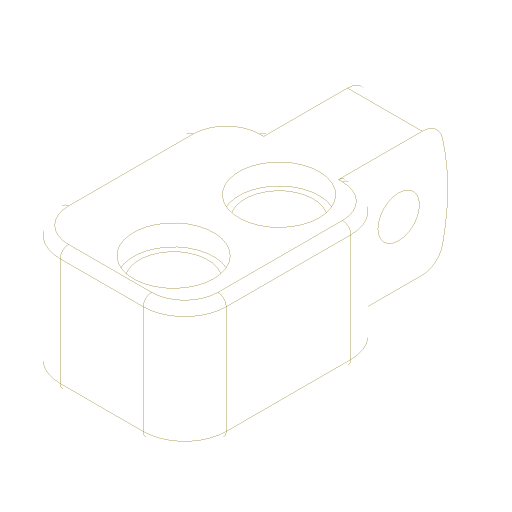
# Autodesk Inventor part: Camera_holder_PCB_1DOF
Saved by Autodesk Inventor 2023 (Build 270158000, 158)
## iProperties
Created: 2024-06-13
Part Number: Camera_holder_PCB_1DOF
Material: Generic
Document SubType Name: Modeling
Designer: ferrerx
Density: 1 g/cm^3
Appearance: Nylon 6
Author: ferrerx
Autodesk Inventor part; units mm, degrees
ref_plane "YZ Plane" through (0, 0, 0) normal (1, 0, 0) x (0, 1, 0)
ref_plane "XZ Plane" through (0, 0, 0) normal (0, 1, 0) x (-1, 0, 0)
ref_plane "XY Plane" through (0, 0, 0) normal (0, 0, 1) x (1, 0, 0)
sketch "Sketch1" plane through (0, 0, 0) normal (0, 1, 0) x (-1, 0, 0)
  line L0 (-2, 2.5) -> (2, 2.5)
  line L1 (2, 2.5) -> (2, -2.5)
  line L2 (2, -2.5) -> (-2, -2.5)
  line L3 (-2, -2.5) -> (-2, 2.5)
  line L4 (-2, 2.5) -> (2, -2.5) construction
  line L5 (2, 2.5) -> (-2, -2.5) construction
  line L6 (0, 0) -> (2, 0) construction
  circle A0 centre (-0.5, 1.27) radius 0.825
  line L7 (-0.5, 1.27) -> (-0.5, 0) construction
  circle A1 centre (-0.5, -1.27) radius 0.825
  line L8 (-0.5, -1.27) -> (-0.5, 0) construction
  dimension "d0" = 4
  dimension "d1" = 5
  dimension "d3" = 1.65
  dimension "d4" = 1.27
  dimension "d5" = 1.5
  constraints: 18 end point, 3 midpoint, 2 centre point, 2 parallel, 1 horizontal, 1 perpendicular, 1 symmetric about line, 1 vertical, 1 other
  measures "d0" distance of L1.end L2.end
  measures "d1" distance of L0.end L1.end
  measures "d3" diameter of A0
  measures "d4" distance from line of L6 L7.start
  measures "d5" distance between parallel lines of L3 L7
extrude "Extrusion1" add sketch "Sketch1" along normal blind 3
sketch "Sketch2" plane through (0, 3, 0) normal (0, 1, 0) x (1, 0, 0)
  circle A0 centre (0.5, -1.27) radius 0.825 projected
  circle A1 centre (0.5, -1.27) radius 0.965
  circle A2 centre (0.5, 1.27) radius 0.825 projected
  circle A3 centre (0.5, 1.27) radius 0.965
  point P0 (0, 0)
  dimension "d8" = 1.93
  dimension "d9" = 1.93
  constraints: 2 centre point, 2 coincident
  measures "d8" diameter of A1
  measures "d9" diameter of A3
extrude "Extrusion2" cut sketch "Sketch2" against normal blind 0.5
sketch "Sketch3" plane through (0, 3, 0) normal (0, 1, 0) x (1, 0, 0)
  line L0 (2, 2.5) -> (-2, 2.5) projected
  line L1 (-0.9, 2.5) -> (0.9, 2.5)
  line L2 (0.9, 2.5) -> (0.9, 5)
  line L3 (0.9, 5) -> (-0.9, 5)
  line L4 (-0.9, 5) -> (-0.9, 2.5)
  line L5 (-2, -2.5) -> (2, -2.5) projected
  line L6 (0, -2.5) -> (0, 2.5) construction
  point P0 (0, 0)
  dimension "d12" = 2.5
  dimension "d13" = 1.8
  constraints: 10 end point, 2 midpoint, 2 parallel, 1 horizontal, 1 perpendicular, 1 point on line, 1 vertical
  measures "d12" distance of L3.end L1.start
  measures "d13" distance between parallel lines of L2 L4
extrude "Extrusion3" add sketch "Sketch3" against normal up to surface (3 mm away)
sketch "Sketch4" plane through (0.9, 3, -2.5) normal (1, 0, 0) x (0, 0, -1)
  line L0 (2.2, 0) -> (2.2, -3) construction
  arc A0 (2.2, -3) -> (2.2, 0) centre (-2.5697, -1.5) ccw
  line L1 (2.5, 0) -> (2.5, -3) projected
  line L2 (2.2, 0) -> (2.5, 0)
  line L3 (2.5, 0) -> (2.5, -3)
  line L4 (2.5, -3) -> (2.2, -3)
  line L5 (2.5, -1.5) -> (1.25, -1.5) construction
  circle A1 centre (1.25, -1.5) radius 0.5
  point P0 (-2.5, -3)
  dimension "d16" = 5
  dimension "d17" = 0.3
  dimension "d18" = 1
  dimension "d19" = 1.25
  constraints: 10 end point, 2 centre point, 2 horizontal, 2 point on circle, 1 coincident, 1 collinear, 1 midpoint, 1 perpendicular, 1 vertical
  measures "d16" radius of A0
  measures "d17" distance between parallel lines of L0 L1
  measures "d18" diameter of A1
  measures "d19" distance of L5.start L5.end
extrude "Extrusion4" cut sketch "Sketch4" against normal blind 10
fillet "Fillet1" radius 0.5 2 edges at (0, 3, -4.7) (0, 0, -4.7)
fillet "Fillet2" radius 1 4 edges at (2, 1.5, -2.5) (2, 1.5, 2.5) (-2, 1.5, -2.5) (-2, 1.5, 2.5)
fillet "Fillet3" radius 0.2 18 edges at (2, 3, 0) (1.7071, 3, -2.2071) (0.95, 3, -2.5) (1.7071, 3, 2.2071) (0, 3, 2.5) (-1.7071, 3, 2.2071) (-2, 3, 0) (-1.7071, 3, -2.2071) (-0.95, 3, -2.5) (1.7071, 0, -2.2071) (0.95, 0, -2.5) (1.7071, 0, 2.2071) (0, 0, 2.5) (-1.7071, 0, 2.2071) (-2, 0, 0) (-1.7071, 0, -2.2071) (-0.95, 0, -2.5) (2, 0, 0)
equation "\"d9\" = d8"
body "Solid1"
